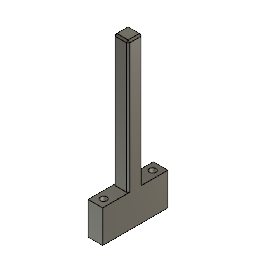
Inner key (Autodesk Fusion 360 design; units mm, degrees)
Autodesk Fusion 360 part; units mm, degrees
sketch "Sketch1" plane through (0, 0, 0) normal (0, 0, 1) x (1, 0, 0)
  circle A0 centre (0, 0) radius 12.5
  circle A1 centre (0, 0) radius 7.5
  line L0 (0, 18) -> (0, -21)
  line L1 (2.25, 6.75) -> (-2.25, 6.75)
  line L2 (-2.25, 6.75) -> (-2.25, -6.75)
  line L3 (-2.25, -6.75) -> (2.25, -6.75)
  line L4 (2.25, -6.75) -> (2.25, 6.75)
  line L5 (2.25, 6.75) -> (-2.25, -6.75) construction
  line L6 (-2.25, 6.75) -> (2.25, -6.75) construction
  circle A2 centre (0, 7.5) radius 1
  circle A3 centre (0, -7.5) radius 1
  line L7 (2.25, -6.75) -> (-2.25, -6.75)
  line L8 (-2.25, -6.75) -> (-2.25, -10.0324)
  line L9 (-2.25, -10.0324) -> (2.25, -10.0324)
  line L10 (2.25, -10.0324) -> (2.25, -6.75)
  line L11 (-2.25, 6.75) -> (2.25, 6.75)
  line L12 (2.25, 6.75) -> (2.25, 9.9416)
  line L13 (2.25, 9.9416) -> (-2.25, 9.9416)
  line L14 (-2.25, 9.9416) -> (-2.25, 6.75)
  dimension "d1" = 25
  dimension "d2" = 15
  dimension "d4" = 2
  dimension "d5" = 2
  dimension "d8" = 4.5
  measures "d1" diameter of A0
  measures "d2" diameter of A1
  measures "d4" diameter of A2
  measures "d5" diameter of A3
  measures "d8" distance of L2 L4
extrude "Extrude2" add sketch "Sketch1" along normal blind 10 contours A1 L0 A2 L12 L13 | A1 L0 A2 L13 L14 | A1 L0 A3 L8 L9 | A1 L0 A3 L9 L10 | A1 L1 A2 L11 L14 | A1 L1 A2 L11 L12 | A1 L3 A3 L7 L8 | A1 L3 A3 L7 L10 | L0 L1 L2 L3 A2 A3 L7 L11 | L0 L1 L3 L4 A2 A3 L7 L11 makes body 1
extrude "Extrude1" add sketch "Sketch1" along normal blind 10 separate body contours L0 L1 L2 L3 A2 A3 L7 L11 | L0 L1 L3 L4 A2 A3 L7 L11 makes body 2
sketch "Sketch3" plane through (0, 0, 10) normal (0, 0, 1) x (-1, 0, 0)
  circle A0 centre (0, -7.5) radius 1
  circle A1 centre (0, 7.5) radius 1
  line L0 (2.25, -9.9416) -> (2.25, 10.0324)
  line L1 (2.25, 10.0324) -> (-2.25, 10.0324)
  line L2 (-2.25, 10.0324) -> (-2.25, -9.9416)
  line L3 (-2.25, -9.9416) -> (2.25, -9.9416)
  line L4 (-2.25, -2.25) -> (2.25, -2.25)
  line L5 (2.25, -2.25) -> (2.25, 2.25)
  line L6 (2.25, 2.25) -> (-2.25, 2.25)
  line L7 (-2.25, 2.25) -> (-2.25, -2.25)
  line L8 (-2.25, -2.25) -> (2.25, 2.25) construction
  line L9 (2.25, -2.25) -> (-2.25, 2.25) construction
  dimension "d11" = 4.5
extrude "Extrude3" add sketch "Sketch3" along normal blind 40 contours L0 L2 L4 L5 L6 L7 bodies 1 2
chamfer "Chamfer1" distance 0.5 angle 45 8 edges at (2.25, 0, 50) (-2.25, 0, 50) (0, -2.25, 50) (0, 2.25, 50) (2.25, 2.25, 30) (-2.25, 2.25, 30) (-2.25, -2.25, 30) (2.25, -2.25, 30) on bodies 1
